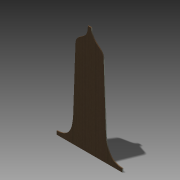
# Autodesk Inventor part: Bottom Plate v1
Saved by Autodesk Inventor 2012 (Build 160160000, 160)
## iProperties
Created: 2013-02-28
Part Number: Bottom Plate v1
Material: Wood (Cherry)
Document SubType Name: Modeling
Designer: fixer
Mass: 71.9783 g
Surface Area: 944.06 cm^2
Volume: 143.957 cm^3
Density: 0.5 g/cm^3
Author: fixer
Autodesk Inventor part; units mm, degrees
ref_plane "YZ Plane" through (0, 0, 0) normal (1, 0, 0) x (0, 1, 0)
ref_plane "XZ Plane" through (0, 0, 0) normal (0, 1, 0) x (-1, 0, 0)
ref_plane "XY Plane" through (0, 0, 0) normal (0, 0, 1) x (1, 0, 0)
sketch "Sketch1" plane through (0, 0, 0) normal (0, 0, 1) x (1, 0, 0)
  line L0 (76.2, -12.7) -> (381, -12.7) construction
  line L1 (-76.2, -12.7) -> (-381, -12.7) construction
  line L2 (-76.2, 0) -> (-381, 0) construction
  line L3 (76.2, 0) -> (381, 0) construction
  line L4 (0, -116.2267) -> (0, 608.4603)
  line L5 (0, -12.7) -> (-114.6099, -12.7)
  line L6 (-114.6099, -12.7) -> (-114.6099, 0)
  line L7 (0, 394.3626) -> (-6.35, 394.3626)
  line L8 (-40.2136, 308.3016) -> (-57.305, 93.11)
  spline S0 degree 3 poles (-114.6099, 0) (-60.3377, 0) (-60.3484, 54.7909) (-57.305, 93.11) knots 0 0 0 0 1 1 1 1
  line L9 (-119.6474, 0) -> (-109.5725, 0) construction
  arc A0 (-118.6349, 0.1005) -> (-110.585, 0.1005) centre (-114.6099, 80.6377) ccw construction
  line L10 (40.2136, 308.3016) -> (57.305, 93.11)
  line L11 (0, 394.3626) -> (6.35, 394.3626)
  spline S1 degree 3 poles (114.6099, 0) (60.3377, 0) (60.3484, 54.7909) (57.305, 93.11) knots 0 0 0 0 1 1 1 1
  line L12 (119.6474, 0) -> (109.5725, 0) construction
  arc A1 (110.585, 0.1005) -> (118.6349, 0.1005) centre (114.6099, 80.6377) ccw construction
  line L13 (0, -12.7) -> (114.6099, -12.7)
  line L14 (114.6099, -12.7) -> (114.6099, 0)
  spline S2 degree 4 poles (-6.35, 394.3626) (-6.35, 372.6715) (-17.579, 345.2739) (-20.8089, 340.9314) (-39.3875, 318.7028) (-40.2136, 308.3016) knots 0 0 0 0 0 0.523271 1 1 1 1 1
  line L15 (-6.35, 421.2444) -> (-6.35, 367.4808) construction
  arc A2 (-8.4521, 373.2806) -> (-8.4521, 415.4446) centre (-113.1163, 394.3626) ccw construction
  spline S3 degree 4 poles (6.35, 394.3626) (6.35, 352.9097) (13.7895, 346.0085) (38.4808, 330.1195) (40.2136, 308.3016) knots 0 0 0 0 0 1 1 1 1 1
  line L16 (6.35, 421.2444) -> (6.35, 367.4808) construction
  arc A3 (8.4521, 415.4446) -> (8.4521, 373.2806) centre (113.1163, 394.3626) ccw construction
  line L17 (-14.8603, 351.5845) -> (-28.3954, 331.1958) construction
  arc A4 (-27.429, 333.5531) -> (-16.6575, 349.7787) centre (-101.0508, 394.1155) ccw construction
  point P0 (0, 0)
  point P1 (-21.6278, 341.3901)
  point P2 (21.6278, 341.3901)
  dimension "d0" = 6.35
  constraints: 36 end point, 16 symmetric about line, 9 horizontal, 8 midpoint, 5 centre point, 5 point on circle, 5 point on line, 4 vertical, 2 perpendicular, 21 other
  measures "d0" distance of L7.start L7.end
extrude "Extrusion1" add sketch "Sketch1" against normal blind 3.175
body "Solid1"
